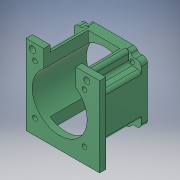
# Autodesk Inventor part: КВ33.000.107 - Крепеж мотора
Saved by Autodesk Inventor 2019 (Build 230136000, 136)
## iProperties
Created: 2021-03-22
Part Number: КВ33.000.107 - Крепеж мотора
Material: PC/ABS Plastic
Document SubType Name: Modeling
Designer: Петров Иван
Density: 0.357273 g/cm^3
Appearance: Smooth - Dark Sea Green
Author: Петров Иван
Autodesk Inventor part; units mm, degrees
ref_plane "YZ Plane" through (0, 0, 0) normal (1, 0, 0) x (0, 1, 0)
ref_plane "XZ Plane" through (0, 0, 0) normal (0, 1, 0) x (-1, 0, 0)
ref_plane "XY Plane" through (0, 0, 0) normal (0, 0, 1) x (1, 0, 0)
sketch "Sketch1" plane through (0, 0, 0) normal (0, 0, 1) x (1, 0, 0)
  line L0 (-17, 21) -> (-21, 17) projected
  line L1 (-21, 17) -> (-21, -17) projected
  line L2 (-21, -17) -> (-17, -21) projected
  line L3 (-17, -21) -> (17, -21) projected
  line L4 (17, -21) -> (21, -17) projected
  line L5 (21, -17) -> (21, 17) projected
  line L6 (21, 17) -> (17, 21) projected
  line L7 (17, 21) -> (-17, 21) projected
  circle A0 centre (-15.5, -15.5) radius 1.5 projected
  circle A1 centre (15.5, -15.5) radius 1.5 projected
  circle A2 centre (15.5, 15.5) radius 1.5 projected
  circle A3 centre (-15.5, 15.5) radius 1.5 projected
  circle A4 centre (0, 0) radius 11 projected
  circle A5 centre (0, 0) radius 17.2047
  point P0 (0, 0)
  constraints: 1 centre point, 1 coincident
extrude "Extrusion1" add sketch "Sketch1" along normal blind 34 contours L7 L6 L5 L4 L3 L2 L1 L0
sketch "Sketch2" plane through (0, 0, 34) normal (0, 0, 1) x (1, 0, 0)
  line L0 (-21, 21) -> (-13.3553, 21)
  line L1 (-13.3553, 21) -> (-13.3553, 13.3468)
  line L2 (-13.3553, 13.3468) -> (-21, 13.3468)
  line L3 (-21, 13.3468) -> (-21, 21)
  point P0 (0, 0)
  point P1 (-17, 21)
  constraints: 8 end point, 2 parallel, 1 horizontal, 1 perpendicular, 1 point on line
extrude "Extrusion2" cut sketch "Sketch2" against normal blind 30
pattern_circular "Circular Pattern2" count 4 over 360 about axis through (0, 0, 0) along (0, 0, 1) of "Extrusion2"
sketch "Sketch3" plane through (-17, 21, 0) normal (0, 1, 0) x (1, 0, 0)
  line L0 (7, -30.7457) -> (27, -30.7457)
  line L1 (27, -30.7457) -> (27, -6.1481)
  line L2 (27, -6.1481) -> (7, -6.1481)
  line L3 (7, -6.1481) -> (7, -30.7457)
  line L4 (17, 0) -> (17, 3.4981)
  dimension "d11" = 10
  constraints: 10 end point, 2 parallel, 1 horizontal, 1 perpendicular, 1 vertical, 1 other
  measures "d11" distance from line of L4.start L3
extrude "Extrusion3" cut sketch "Sketch3" against normal blind 9
fillet "Fillet2" radius 2 12 edges at (-13.3553, 13.3468, 19) (-21, 13.3468, 19) (-13.3553, 21, 19) (13.3468, 21, 19) (13.3468, 13.3553, 19) (21, 13.3553, 19) (21, -13.3468, 19) (13.3553, -13.3468, 19) (13.3553, -21, 19) (-13.3468, -21, 19) (-13.3468, -13.3553, 19) (-21, -13.3553, 19)
pattern_circular "Circular Pattern3" count 2 over 360 about axis through (0, 0, 0) along (0, 0, 1) of "Extrusion3"
sketch "Sketch4" plane through (0, 0, 34) normal (0, 0, 1) x (1, 0, 0)
  line L0 (-25, -25) -> (25, -25)
  line L1 (25, -25) -> (25, 25)
  line L2 (25, 25) -> (-25, 25)
  line L3 (-25, 25) -> (-25, -25)
  line L4 (-25, -25) -> (25, 25) construction
  line L5 (25, -25) -> (-25, 25) construction
  circle A0 centre (0, 0) radius 17.2047 projected
  point P0 (0, 0)
  dimension "d18" = 50
  dimension "d19" = 50
  constraints: 12 end point, 2 midpoint, 2 parallel, 1 horizontal, 1 perpendicular
  measures "d18" distance of L2.end L1.end
  measures "d19" distance of L1.end L0.end
extrude "Extrusion4" add sketch "Sketch4" against normal blind 4
sketch "Sketch5" plane through (-25, 25, 34) normal (0, 1, 0) x (1, 0, 0)
  line L0 (15, 4) -> (35, 4) projected
  line L1 (0, 0) -> (50, 0) projected
  line L2 (35, 4) -> (14.6906, 4)
  line L3 (14.3224, 0) -> (35, 0)
  line L4 (35, 0) -> (35, 4)
  line L5 (15, 4) -> (15, 27.8519) projected
  line L6 (15, 4) -> (15, 0)
  point P0 (25, 34)
  constraints: 8 end point, 2 point on line, 1 horizontal, 1 parallel, 1 perpendicular
extrude "Extrusion5" cut sketch "Sketch5" against normal blind 22.5
sketch "Sketch7" plane through (0, 0, 30) normal (0, 0, -1) x (-1, 0, 0)
  line L0 (-25, -25) -> (25, -25) projected
  line L1 (25, 25) -> (25, -25) projected
  line L2 (21, -25) -> (25, -25)
  line L3 (25, -25) -> (25, 25)
  line L4 (25, 25) -> (21, 25)
  line L5 (21, 25) -> (21, -25)
  line L6 (21, 17) -> (21, -17) projected
  point P0 (0, 0)
  point P1 (10, -25)
  point P2 (21, 0)
  constraints: 8 end point, 2 midpoint, 2 parallel, 1 horizontal, 1 perpendicular, 1 point on line
extrude "Extrusion6" cut sketch "Sketch7" against normal blind 60.5
sketch "Sketch8" plane through (0, 0, 30) normal (0, 0, -1) x (-1, 0, 0)
  circle A0 centre (-17, 21) radius 2
  line L0 (-10, 25) -> (-25, 25) projected
  line L1 (-25, 25) -> (-25, -25) projected
  point P0 (0, 0)
  dimension "d27" = 4
  dimension "d28" = 4
  dimension "d29" = 8
  constraints: 1 centre point
  measures "d27" diameter of A0
  measures "d28" distance from line of L0 A0.centre
  measures "d29" distance from line of L1 A0.centre
extrude "Extrusion7" cut sketch "Sketch8" against normal blind 60.5
sketch "Sketch9" plane through (0, 0, 30) normal (0, 0, -1) x (-1, 0, 0)
  circle A0 centre (17, 21) radius 2
  line L0 (21, 11.3468) -> (21, 25) projected
  line L1 (21, 25) -> (10, 25) projected
  point P0 (0, 0)
  dimension "d32" = 4
  dimension "d33" = 4
  dimension "d34" = 4
  constraints: 1 centre point
  measures "d32" diameter of A0
  measures "d33" distance from line of L0 A0.centre
  measures "d34" distance from line of L1 A0.centre
extrude "Extrusion8" cut sketch "Sketch9" against normal blind 6.5
fillet "Fillet4" radius 2.75 4 edges at (-17, 21, 2) (-17, -21, 2) (17, -21, 2) (17, 21, 2) inverted yes
fillet "Fillet5" radius 2.75 12 edges at (-14.25, 21, 2) (-18.9445, 19.0555, 2) (-18.9445, -19.0555, 2) (-14.25, -21, 2) (-21, 17, 2) (-21, -17, 2) (18.9445, 19.0555, 2) (14.25, 21, 2) (18.9445, -19.0555, 2) (14.25, -21, 2) (21, -17, 2) (21, 17, 2)
sketch "Sketch11" plane through (0, 0, 34) normal (0, 0, 1) x (1, 0, 0)
  circle A0 centre (-15.5, 15.5) radius 1.5 projected
  circle A1 centre (-15.5, -15.5) radius 1.5 projected
  circle A2 centre (15.5, 15.5) radius 1.5 projected
  circle A3 centre (15.5, -15.5) radius 1.5 projected
  point P0 (0, 0)
extrude "Extrusion10" cut sketch "Sketch11" against normal blind 8.5
body "Solid1"
